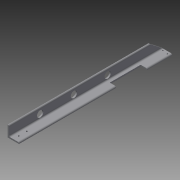
# Autodesk Inventor part: 2x2 quarter in angle aluminum far side
Saved by Autodesk Inventor 2015 (Build 190159000, 159)
## iProperties
Created: 2015-02-01
Part Number: 2x2 quarter in angle aluminum far side
Material: Generic
Document SubType Name: Modeling
Designer: szymsea16
Density: 1 g/cm^3
Appearance: Default
Author: szymsea16
Autodesk Inventor part; units mm, degrees
ref_plane "YZ Plane" through (0, 0, 0) normal (1, 0, 0) x (0, 1, 0)
ref_plane "XZ Plane" through (0, 0, 0) normal (0, 1, 0) x (-1, 0, 0)
ref_plane "XY Plane" through (0, 0, 0) normal (0, 0, 1) x (1, 0, 0)
sketch "Sketch1" plane through (0, 0, 0) normal (0, 1, 0) x (-1, 0, 0)
  line L0 (0, 0) -> (50.8, 0)
  line L1 (50.8, 0) -> (50.8, -736.6)
  line L2 (50.8, -736.6) -> (0, -736.6)
  line L3 (0, -736.6) -> (0, 0)
  dimension "d0" = 50.8
  dimension "d1" = 736.6
  constraints: 8 end point, 2 horizontal, 1 parallel, 1 perpendicular
  measures "d0" distance of L0.start L0.end
  measures "d1" distance of L0.end L1.end
extrude "Extrusion1" add sketch "Sketch1" along normal blind 6.35
sketch "Sketch2" plane through (0, 6.35, 0) normal (0, 1, 0) x (1, 0, 0)
  line L0 (-50.8, 0) -> (-44.45, 0)
  line L1 (-50.8, 0) -> (0, 0) projected
  line L2 (-44.45, 0) -> (-44.45, 736.6)
  line L3 (0, 736.6) -> (-50.8, 736.6) projected
  line L4 (-44.45, 736.6) -> (-50.8, 736.6)
  line L5 (-50.8, 736.6) -> (-50.8, 0)
  line L6 (-50.8, 0) -> (-44.45, 0)
  dimension "d4" = 6.35
  dimension "d5" = 736.6
  dimension "d6" = 736.6
  constraints: 10 end point, 1 perpendicular, 1 point on line, 1 vertical
  measures "d4" distance of L0.start L0.end
  measures "d5" distance of L0.end L2.end
  measures "d6" distance of L3.end L0.start
extrude "Extrusion2" add sketch "Sketch2" along normal blind 44.45
fillet "Fillet1" radius 6.35 1 edges at (-44.45, 6.35, -368.3)
fillet "Fillet2" radius 6.35 1 edges at (0, 6.35, -368.3)
fillet "Fillet3" radius 6.35 1 edges at (-44.45, 50.8, -368.3)
hole "Hole1" at (-44.45, 25.4, -184.15) direction (-1, 0, 0) diameter 14.605 end through all
pattern_linear "Rectangular Pattern1" count 3 spacing 152.4 along (0, 0, -1) of "Hole1"
sketch "Sketch4" plane through (-44.45, 12.7, 0) normal (1, 0, 0) x (0, 0, -1)
  line L0 (43.5102, 15.9813) -> (43.5102, 68.613)
  line L1 (43.5102, 68.613) -> (43.5102, -117.0764)
  line L2 (43.5102, -117.0764) -> (-179.7757, -29.554)
  line L3 (-179.7757, -29.554) -> (-128.9181, 50.2806)
  line L4 (-128.9181, 50.2806) -> (-52.0403, 93.4505)
  line L5 (-52.0403, 93.4505) -> (43.5102, 68.613)
  point P0 (0, -12.7)
  constraints: 12 end point, 1 point on line
extrude "Extrusion3" cut sketch "Sketch4" along normal through all both and the other way through all
sketch "Sketch6" plane through (-50.8, 0, -736.6) normal (-1, 0, 0) x (0, 0, 1)
  line L0 (0, 0) -> (31.75, 0)
  line L1 (693.0898, 0) -> (0, 0) projected
  line L2 (31.75, 0) -> (31.75, 50.8)
  line L3 (0, 50.8) -> (693.0898, 50.8) projected
  line L4 (0, 0) -> (0, 19.05)
  line L5 (0, 0) -> (0, 50.8) projected
  line L6 (0, 19.05) -> (31.75, 50.8)
  line L7 (31.75, 87.3968) -> (-26.0736, 76.8736)
  line L8 (-26.0736, 76.8736) -> (-32.5199, 38.9128)
  line L9 (-32.5199, 38.9128) -> (0, 19.05)
  line L10 (31.75, 87.3968) -> (31.75, 50.8)
  point P0 (736.6, 0)
  dimension "d38" = 31.75
  dimension "d39" = 19.05
  constraints: 16 end point, 4 point on line, 2 perpendicular
  measures "d38" distance of L0.start L0.end
  measures "d39" distance of L0.start L4.end
extrude "Extrusion4" cut sketch "Sketch6" against normal blind 304.8 contours L5 L3 L6
sketch "Sketch7" plane through (-50.8, 0, -736.6) normal (-1, 0, 0) x (0, 0, 1)
  line L0 (0, 0) -> (0, 6.35)
  line L1 (0, 0) -> (0, 19.05) projected
  line L2 (0, 6.35) -> (0, 61.7609)
  line L3 (0, 61.7609) -> (31.75, 50.8)
  line L4 (31.75, 50.8) -> (57.15, 50.8)
  line L5 (31.75, 50.8) -> (693.0898, 50.8) projected
  line L6 (57.15, 50.8) -> (0, 6.35)
  point P0 (736.6, 0)
  dimension "d42" = 6.35
  dimension "d43" = 25.4
  constraints: 10 end point, 3 point on line
  measures "d42" distance of L0.start L0.end
  measures "d43" distance of L3.end L4.end
extrude "Extrusion5" cut sketch "Sketch7" against normal blind 304.8
sketch "Sketch10" plane through (0, 6.35, 0) normal (0, 1, 0) x (1, 0, 0)
  circle A0 centre (-10.8427, 725.424) radius 2.667
  circle A1 centre (-33.7027, 727.71) radius 2.667
  point P0 (0, 0)
  constraints: 2 centre point, 4 other
extrude "Extrusion6" cut sketch "Sketch10" against normal blind 25.4
sketch "Sketch12" plane through (-50.8, 0, -736.6) normal (-1, 0, 0) x (0, 0, 1)
  circle A0 centre (400.05, 25.4) radius 7.3025 projected
  circle A1 centre (552.45, 25.4) radius 7.3025 projected
  circle A2 centre (247.65, 25.4) radius 7.3025 projected
  circle A3 centre (247.65, 25.4) radius 14.2875
  circle A4 centre (400.05, 25.4) radius 14.2875
  circle A5 centre (552.45, 25.4) radius 14.2875
  point P0 (736.6, 0)
  dimension "d48" = 28.575
  dimension "d49" = 28.575
  dimension "d50" = 28.575
  constraints: 3 centre point, 3 coincident
  measures "d48" diameter of A3
  measures "d49" diameter of A4
  measures "d50" diameter of A5
extrude "Extrusion7" cut sketch "Sketch12" against normal blind 25.4
sketch "Sketch13" plane through (0, 6.35, 0) normal (0, 1, 0) x (1, 0, 0)
  circle A0 centre (-25.4, 68.2719) radius 3.175
  circle A1 centre (-25.4, 104.4702) radius 3.175
  point P0 (0, 0)
  constraints: 2 centre point, 4 other
extrude "Extrusion8" cut sketch "Sketch13" against normal blind 25.4
sketch "Sketch14" plane through (0, 6.35, 0) normal (0, 1, 0) x (1, 0, 0)
  circle A0 centre (-25.4, 68.2719) radius 3.175 projected
  circle A1 centre (-25.4, 104.4702) radius 3.175 projected
  circle A2 centre (-10.8427, 725.424) radius 2.667 projected
  circle A3 centre (-33.7027, 727.71) radius 2.667 projected
  line L0 (-38.1, 43.5102) -> (-6.35, 43.5102) projected
  line L1 (-6.35, 736.6) -> (-6.35, 43.5102) projected
  line L2 (-6.35, 736.6) -> (-38.1, 736.6) projected
  line L3 (-38.1, 43.5102) -> (-38.1, 736.6) projected
  line L4 (-6.35, 43.5102) -> (0, 43.5102) projected
  line L5 (0, 736.6) -> (0, 43.5102) projected
  line L6 (0, 736.6) -> (-6.35, 736.6) projected
  line L7 (-6.35, 736.6) -> (-6.35, 43.5102) projected
  line L8 (11.781, 501.9003) -> (-12.6385, 502.7611)
  line L9 (-13.1288, 510.961) -> (-13.1288, 506.3701)
  line L10 (-13.1288, 503.6795) -> (-13.1288, 506.3701)
  ellipse E0 centre (-12.6208, 503.2688) end of major axis (-12.1128, 503.2688) minor radius 0.508 (-13.1288, 503.2688) -> (-12.6385, 502.7611) ccw
  line L11 (-13.1288, 518.5072) -> (-13.1288, 510.961)
  line L12 (-13.1288, 526.3619) -> (-13.1288, 520.4519)
  line L13 (-13.1288, 518.5844) -> (-13.1288, 520.4519)
  line L14 (-21.3838, 525.728) -> (-6.0168, 525.728)
  line L15 (-21.3838, 530.5032) -> (-21.3838, 525.728)
  line L16 (-21.3838, 530.5032) -> (-6.0168, 530.5032)
  line L17 (-13.9225, 584.3659) -> (-13.9225, 520.3579)
  line L18 (-15.6688, 579.6293) -> (-15.6688, 550.0287)
  line L19 (-21.8918, 577.0337) -> (-21.8918, 580.7929)
  line L20 (-15.6688, 589.4756) -> (-15.6688, 583.2973)
  line L21 (-14.1739, 593.5184) -> (5.7789, 610.1541)
  line L22 (-13.4799, 597.3719) -> (6.1422, 615.7328)
  line L23 (0, 736.6) -> (0, 43.5102) projected
  line L24 (0, 482.6) -> (-28.575, 482.6)
  line L25 (-28.575, 482.6) -> (-28.575, 622.3)
  line L26 (-28.575, 622.3) -> (0, 622.3)
  line L27 (0, 622.3) -> (0, 482.6)
  point P0 (0, 0)
  dimension "d55" = 139.7
  constraints: 38 end point, 10 vertical, 3 horizontal, 2 parallel, 1 perpendicular, 1 point on line, 35 other
  measures "d55" distance of L24.end L25.end
extrude "Extrusion9" cut sketch "Sketch14" against normal blind 6.35 contours L24 L25 L26 L1 L16 L15 L14 | L1 L8 L5 L24 | L1 L21 L5 L8 | L26 L5 L22 L1 | L14 L17 L16 L1 | L22 L5 L21 L1 | L17 L14 L15 L16
body "Solid1"
